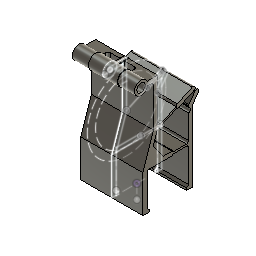
Camera_suporte_Complient_mechanism v2 (Autodesk Fusion 360 design; units mm, degrees)
Autodesk Fusion 360 part; units mm, degrees
sketch "Sketch1" plane through (0, 0, 0) normal (1, 0, 0) x (0, 1, 0)
  line L0 (-10, 18) -> (10, 18) construction
  line L1 (10, 18) -> (10, 0) construction
  line L2 (10, 0) -> (-10, 0) construction
  line L3 (-10, 0) -> (-10, 18) construction
  line L4 (-10, 18) -> (-5, 33)
  line L5 (-5, 33) -> (-5, 55.3246)
  line L6 (-5, 55.3246) -> (-13, 55.3246)
  circle A0 centre (-13, 54.0746) radius 1.25
  circle A1 centre (-13, 54.0746) radius 3.25
  line L7 (10, 18) -> (12, 18)
  line L8 (12, 18) -> (12, 0)
  line L9 (12, 0) -> (10, 0)
  line L10 (10, 0) -> (10, 18)
  line L11 (10, 18) -> (-10, 18) construction
  line L12 (-10, 0) -> (-12.1082, 0)
  line L13 (-12.1082, 0) -> (-12.1082, 18)
  line L14 (-12.1082, 18) -> (-10, 18)
  line L15 (-10, 18) -> (-10, 0)
  line L16 (-12.1082, 18) -> (-7, 33.3246)
  line L17 (-7, 33.3246) -> (-7, 53.3246)
  line L18 (-7, 53.3246) -> (-15.5, 53.3246)
  line L19 (-10, 18) -> (2, 18)
  line L20 (2, 18) -> (2, 20)
  line L21 (2, 20) -> (-10, 20)
  line L22 (-10, 20) -> (-10, 18)
  line L23 (-5, 45.3246) -> (-7, 45.3246)
  line L24 (-7, 53.3246) -> (-7, 55.3246)
  line L25 (1.5, 19) -> (11.5, 19)
  line L26 (-5, 33) -> (12.2198, 41.0297)
  circle A2 centre (-5, 33) radius 19 construction
  line L27 (11.7972, 41.9361) -> (4.5468, 38.5551)
  arc A3 (4.5468, 38.5551) -> (5.392, 36.7425) centre (4.9694, 37.6488) ccw
  line L28 (5.392, 36.7425) -> (12.6425, 40.1234)
  arc A4 (12.6425, 40.1234) -> (11.7972, 41.9361) centre (12.2198, 41.0297) ccw
  line L29 (12.2198, 41.0297) -> (4.9694, 37.6488) construction
  circle A5 centre (10, 33) radius 1
  line L30 (10, 18) -> (10, 38)
  line L31 (10, 38) -> (12, 38)
  line L32 (12, 38) -> (12, 18)
  line L33 (12, 18) -> (10, 18)
  line L34 (10, 35.2) -> (12, 38)
  line L35 (12, 38) -> (13.7437, 40.4412)
  line L36 (13.7437, 40.4412) -> (15.3712, 39.2787)
  line L37 (15.3712, 39.2787) -> (12, 34.5591)
  line L38 (10, 0) -> (9, 0)
  line L39 (9, 0) -> (9, 1)
  line L40 (9, 1) -> (10, 1)
  line L41 (10, 1) -> (10, 0)
  line L42 (9, 1) -> (10, 2)
  line L43 (0, 0) -> (0, -6.8646) construction
  line L44 (-10, 1) -> (-10, 0)
  line L45 (-9, 1) -> (-10, 1)
  line L46 (-9, 1) -> (-10, 2)
  line L47 (-9, 0) -> (-9, 1)
  line L48 (-10, 0) -> (-9, 0)
  circle A6 centre (-5, 33) radius 15 construction
  point P0 (2, 19)
  dimension "d1" = 20
  dimension "d2" = 18
  dimension "d3" = 15
  dimension "d5" = 8
  dimension "d6" = 5
  dimension "d7" = 2.5
  dimension "d8" = 6.5
  dimension "d9" = 2
  dimension "d31" = 8
  dimension "d48" = 8
  dimension "d62" = 20
  dimension "d63" = 2
  dimension "d106" = 90
  dimension "d109" = 65
  dimension "d110" = 2
  dimension "d111" = 8
  dimension "d124" = 2
  dimension "d125" = 20
  dimension "d126" = 3
  dimension "d127" = 2.8
  dimension "d128" = 1
  dimension "d129" = 45
  dimension "d130" = 1
  dimension "d131" = 0.5
  dimension "d132" = 0.5
  dimension "d134" = 4
  constraint horizontal L0
  constraint horizontal L2
  constraint vertical L3
  constraint midpoint L43.start L2
  constraint perpendicular L0 L5
  constraint perpendicular L5 L6
  constraint coincident L6.end A0
  constraint vertical L6.end A0.centre
  constraint concentric A0 A1
  constraint perpendicular L7 L8
  constraint parallel L7 L9
  constraint parallel L8 L10
  constraint equal L1 L10
  constraint horizontal L11
  constraint equal L2 L11
  constraint horizontal L12
  constraint vertical L13
  constraint horizontal L14
  constraint vertical L15
  constraint coincident L13.end L14.start
  constraint coincident L0.start L3.end
  constraint horizontal L19
  constraint vertical L20
  constraint horizontal L21
  constraint vertical L22
  constraint coincident L5 L23.start
  constraint coincident L17 L23.end
  constraint perpendicular L17 L23
  constraint vertical L1
  constraint coincident L6 L24.end
  constraint perpendicular L6 L24
  constraint coincident L4.end L5.start
  constraint coincident L26.end A2
  constraint tangent L27 A3
  constraint tangent A3 L28
  constraint parallel L27 L28
  constraint tangent L28 A4
  constraint tangent L27 A4
  constraint coincident L26 A3.centre
  constraint parallel L26 L29
  constraint coincident L26.end A4.centre
  constraint equal A4 A5
  constraint midpoint L20 P0
  constraint coincident L25 P0
  constraint perpendicular L30 L31
  constraint parallel L30 L32
  constraint parallel L31 L33
  constraint coincident A5.centre L30
  constraint horizontal L4.end A5.centre
  constraint horizontal L25
  constraint coincident L30 L34.start
  constraint parallel L34 L35
  constraint perpendicular L35 L36
  constraint coincident L32 L37.end
  constraint perpendicular L36 L37
  constraint equal L31 L36
  constraint vertical L32
  constraint horizontal L38
  constraint vertical L39
  constraint horizontal L40
  constraint vertical L41
  constraint coincident L10 L42.end
  constraint coincident L43.start origin
  constraint perpendicular L2 L43
  constraint symmetric L1.end L43 L2.end
  constraint symmetric L38.end L43 L47.start
  constraint symmetric L39.end L43 L45.start
  constraint symmetric L40.end L43 L44.start
  constraint symmetric L42.end L43 L46.end
  constraint concentric A2 A6
  constraint coincident A5.centre A6
  measures "d1" distance of L1.end L2.end
  measures "d2" distance of L0.end L1.end
  measures "d3" vertical distance of L0.start L4.end
  measures "d5" distance of L5.end L6.end
  measures "d6" distance of L3 L5
  measures "d7" diameter of A0
  measures "d8" diameter of A1
  measures "d9" distance of L0.end L7.end
  measures "d31" distance of L18 L23
  measures "d48" distance of L0.end L20
  measures "d62" distance of L16.end L17.end
  measures "d63" distance of L11 L21
  measures "d106" angle of L10 L25
  measures "d109" angle of L5 L26
  measures "d110" distance of L27 L28
  measures "d111" distance of L26.end A3.centre
  measures "d124" distance of L30.end L31.end
  measures "d125" distance of L31.end L7.end
  measures "d126" distance of L31.end L35.end
  measures "d127" distance of L31 L34.start
  measures "d128" distance of L10 L39
  measures "d129" angle of L40 L42
  measures "d130" distance of L38.end L39.end
  measures "d131" distance of L25.end L32
  measures "d132" distance of L20 L25.start
  measures "d134" distance of A2 A6
extrude "Extrude1" add sketch "Sketch1" along normal mid plane 30 contours L4 L21 L22 | L12 L13 L14 L15 L44 | L4 L19 L20 L21 | L4 L5 L14 L16 L17 L21 L22 L23 | L15 L45 L46 | L15 L44 L45 L47 L48 | L5 L6 L17 L23 L24 | L6 A1 L18 L24 | L6 A0 A1 L18 | L6 A0 A1 L18 | L7 A5 L30 L32 L33 L34 | L7 L8 L9 L10 L33 L41 | L10 L40 L42 | L32 L35 L36 L37 | L10 L38 L39 L40 L41 | L27 A3 L28 A4 makes body 1 at (5, -5, 40.4415) makes body 2 at (-5, 12, 23.0394) makes body 3 at (-5, 7.8088, 37.8695)
extrude "Extrude2" add sketch "Sketch1" along normal up to surface (-15 mm away) and the other way up to surface (-15 mm away) thin wall 0.9 centred open curves L25 L26 bodies 2 3 1
extrude "Extrude16" cut sketch "Sketch1" along normal mid plane 14 contours L6 A1 L18 L24 | L6 A0 A1 L18 | L6 A0 A1 L18 bodies 2
move_face "OffsetFaces2" offset -0.8 1 faces at (12.3333, -11.9022, 54.6724) on bodies 2
extrude "Extrude17" add 1 faces at (5, -4.9366, 32.8641) along direction (0, -0.906308, -0.422618) up to surface end surface through (0, -9.3333, 20) normal (0, 0.948683, -0.316228) offset 0 on bodies 2 bodies 2
fillet "Fillet6" radius 1 14 edges at (-7, -7, 54.3246) (7, -7, 54.3246) (0, 10, 34) (0, 10, 35.2) (0, 13.7437, 40.4412) (0, 15.3712, 39.2787) (0, 2, 19.45) (0, 2, 18.55) (0, -5, 33.4965) (0, -5.196, 32.4121) (0, 10, 18.55) (0, 10, 19.45) (11, -7, 53.3246) (-11, -7, 53.3246) on bodies 2
chamfer "Chamfer4" distance 7 angle 45 1 edges at (0, -9.3333, 20) on bodies 2
extrude "Extrude19" cut sketch "Sketch1" along normal mid plane 2 contours L5 L6 L17 L23 L24 | L6 A1 L18 L24 bodies 2
extrude "Extrude20" add sketch "Sketch1" along normal up to surface (-7 mm away) and the other way up to surface (-7 mm away) thin wall 0.45 centred open curves A0 A1 bodies 2
extrude "Extrude21" add sketch "Sketch1" along normal up to surface (1 mm away) and the other way up to surface (1 mm away) thin wall 0.45 centred open curves L6 bodies 2
equation "d122 = ( 0.6 * 2 ) * 1 mm"
